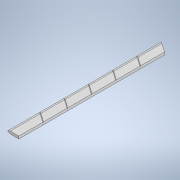
# Autodesk Inventor part: blade a.
Saved by Autodesk Inventor 2021 (Build 250183000, 183)
## iProperties
Created: 2021-03-27
Part Number: blade a.
Material: Generic
Document SubType Name: Modeling
Designer: newic
Density: 1 g/cm^3
Appearance: Default
Author: newic
Autodesk Inventor part; units mm, degrees
ref_plane "YZ Plane" through (0, 0, 0) normal (1, 0, 0) x (0, 1, 0)
ref_plane "XZ Plane" through (0, 0, 0) normal (0, 1, 0) x (-1, 0, 0)
ref_plane "XY Plane" through (0, 0, 0) normal (0, 0, 1) x (1, 0, 0)
sketch "Sketch1" plane through (0, 0, 0) normal (0, 1, 0) x (-1, 0, 0)
  line L0 (0, 0) -> (50.9694, 0)
  line L1 (50.9694, 0) -> (50.9694, -698.5)
  line L2 (0, -662.8108) -> (0, 0)
  line L3 (50.9694, -698.5) -> (133.3543, -698.5) construction
  line L4 (0, -647.5306) -> (0, -662.8108)
  line L5 (0, -662.8108) -> (50.9694, -698.5)
  dimension "d0" = 698.5
  dimension "d10" = 55
  constraints: 12 end point, 2 horizontal, 1 collinear, 1 parallel, 1 perpendicular, 1 point on line
  measures "d0" distance of L0.end L1.end
  measures "d10" angle of L5 L1
extrude "Extrusion1" add sketch "Sketch1" along normal blind 11.43
chamfer "Chamfer1" distance 11.43 angle 22.5 1 edges at (-50.9694, 11.43, -349.25) measured on face at (-33.9796, 11.43, -453.7703)
chamfer "Chamfer2" distance 11.43 angle 22.5 1 edges at (-50.9694, 0, -349.25) measured on face at (-33.9796, 0, -453.7703)
sketch "Sketch2" plane through (0, 11.43, 0) normal (0, 1, 0) x (1, 0, 0)
  line L0 (0, 0) -> (0, 662.8108) projected
  line L1 (0, 662.8108) -> (-39.5394, 690.4966) projected
  line L2 (0, 0) -> (0, 662.8108)
  line L3 (0, 662.8108) -> (0, 552.3208)
  line L4 (0, 552.3208) -> (0, 441.8308)
  line L5 (0, 441.8308) -> (0, 331.3408)
  line L6 (0, 331.3408) -> (0, 220.8508)
  line L7 (0, 220.8508) -> (0, 110.3608)
  line L8 (0, 110.3608) -> (0, -0.1292)
  line L9 (-50.9694, 698.5) -> (-50.9694, 0) projected
  line L10 (0, 552.3208) -> (62.2222, 552.3208) construction
  line L11 (0, 441.8308) -> (75.6755, 441.8308) construction
  line L12 (0, 331.3408) -> (96.3167, 331.3408) construction
  line L13 (0, 220.8508) -> (100.8131, 220.8508) construction
  line L14 (0, 110.3608) -> (129.8585, 110.3608) construction
  line L15 (0.7284, 553.3611) -> (-50.241, 589.0503)
  line L16 (-0.7284, 551.2805) -> (-51.6979, 586.9697)
  line L17 (0.7284, 442.8711) -> (-50.241, 478.5603)
  line L18 (-0.7284, 440.7905) -> (-51.6979, 476.4797)
  line L19 (0.7284, 332.3811) -> (-50.241, 368.0703)
  line L20 (-0.7284, 330.3005) -> (-51.6979, 365.9897)
  line L21 (0.7284, 221.8911) -> (-50.241, 257.5803)
  line L22 (-0.7284, 219.8105) -> (-51.6979, 255.4997)
  line L23 (0.7284, 111.4011) -> (-50.241, 147.0903)
  line L24 (-0.7284, 109.3205) -> (-51.6979, 145.0097)
  line L25 (-55.7095, 150.6945) -> (-51.6979, 145.0097)
  line L26 (6.2736, 109.3205) -> (0.7284, 111.4011)
  line L27 (4.7871, 219.8105) -> (0.7284, 221.8911)
  line L28 (-50.241, 257.5803) -> (-56.0233, 261.6292)
  line L29 (-56.0233, 261.6292) -> (-51.6979, 255.4997)
  line L30 (-0.7284, 109.3205) -> (2.432, 107.1075)
  line L31 (2.432, 107.1075) -> (6.2736, 109.3205)
  line L32 (-50.241, 147.0903) -> (-53.1322, 149.1147)
  line L33 (-53.1322, 149.1147) -> (-55.7095, 150.6945)
  line L34 (-0.7284, 219.8105) -> (1.0647, 218.5549)
  line L35 (1.0647, 218.5549) -> (4.7871, 219.8105)
  line L36 (-0.7284, 330.3005) -> (6.2736, 325.3976)
  line L37 (6.2736, 325.3976) -> (0.7284, 332.3811)
  line L38 (-50.241, 368.0703) -> (-56.0233, 372.1192)
  line L39 (-56.0233, 372.1192) -> (-51.6979, 365.9897)
  line L40 (-0.7284, 440.7905) -> (6.2736, 435.8876)
  line L41 (6.2736, 435.8876) -> (0.7284, 442.8711)
  line L42 (-50.241, 478.5603) -> (-56.4046, 482.8761)
  line L43 (-56.4046, 482.8761) -> (-51.6979, 476.4797)
  line L44 (-0.7284, 551.2805) -> (4.3528, 547.7226)
  line L45 (4.3528, 547.7226) -> (0.7284, 553.3611)
  line L46 (-50.241, 589.0503) -> (-53.8606, 591.5848)
  line L47 (-53.8606, 591.5848) -> (-51.6979, 586.9697)
  dimension "d11" = 110.49
  dimension "d12" = 110.49
  dimension "d13" = 110.49
  dimension "d14" = 110.49
  dimension "d15" = 110.49
  dimension "d16" = 110.49
  constraints: 90 end point, 10 point on line, 8 parallel, 5 horizontal, 1 vertical
  measures "d11" distance of L0.end L3.end
  measures "d12" distance of L3.end L4.end
  measures "d13" distance of L4.end L5.end
  measures "d14" distance of L5.end L6.end
  measures "d15" distance of L6.end L7.end
  measures "d16" distance of L7.end L8.end
sketch "Sketch3" plane through (0, 0, 0) normal (0, -1, 0) x (1, 0, 0)
  line L0 (0, 0) -> (0, 662.8108)
  line L1 (0, 662.8108) -> (-39.5394, 690.4966)
  line L2 (0, 0) -> (0, 662.8108)
  line L3 (0, 662.8108) -> (0, 552.3208)
  line L4 (0, 552.3208) -> (0, 441.8308)
  line L5 (0, 441.8308) -> (0, 331.3408)
  line L6 (0, 331.3408) -> (0, 220.8508)
  line L7 (0, 220.8508) -> (0, 110.3608)
  line L8 (0, 110.3608) -> (0, -0.1292)
  line L9 (-50.9694, 698.5) -> (-50.9694, 0)
  line L10 (0, 552.3208) -> (62.2222, 552.3208) construction
  line L11 (0, 441.8308) -> (75.6755, 441.8308) construction
  line L12 (0, 331.3408) -> (96.3167, 331.3408) construction
  line L13 (0, 220.8508) -> (100.8131, 220.8508) construction
  line L14 (0, 110.3608) -> (129.8585, 110.3608) construction
  line L15 (0.7284, 553.3611) -> (-50.241, 589.0503)
  line L16 (-0.7284, 551.2805) -> (-51.6979, 586.9697)
  line L17 (0.7284, 442.8711) -> (-50.241, 478.5603)
  line L18 (-0.7284, 440.7905) -> (-51.6979, 476.4797)
  line L19 (0.7284, 332.3811) -> (-50.241, 368.0703)
  line L20 (-0.7284, 330.3005) -> (-51.6979, 365.9897)
  line L21 (0.7284, 221.8911) -> (-50.241, 257.5803)
  line L22 (-0.7284, 219.8105) -> (-51.6979, 255.4997)
  line L23 (0.7284, 111.4011) -> (-50.241, 147.0903)
  line L24 (-0.7284, 109.3205) -> (-51.6979, 145.0097)
  line L25 (-55.7095, 150.6945) -> (-51.6979, 145.0097)
  line L26 (6.2736, 109.3205) -> (0.7284, 111.4011)
  line L27 (4.7871, 219.8105) -> (0.7284, 221.8911)
  line L28 (-50.241, 257.5803) -> (-56.0233, 261.6292)
  line L29 (-56.0233, 261.6292) -> (-51.6979, 255.4997)
  line L30 (-0.7284, 109.3205) -> (2.432, 107.1075)
  line L31 (2.432, 107.1075) -> (6.2736, 109.3205)
  line L32 (-50.241, 147.0903) -> (-53.1322, 149.1147)
  line L33 (-53.1322, 149.1147) -> (-55.7095, 150.6945)
  line L34 (-0.7284, 219.8105) -> (1.0647, 218.5549)
  line L35 (1.0647, 218.5549) -> (4.7871, 219.8105)
  line L36 (-0.7284, 330.3005) -> (6.2736, 325.3976)
  line L37 (6.2736, 325.3976) -> (0.7284, 332.3811)
  line L38 (-50.241, 368.0703) -> (-56.0233, 372.1192)
  line L39 (-56.0233, 372.1192) -> (-51.6979, 365.9897)
  line L40 (-0.7284, 440.7905) -> (6.2736, 435.8876)
  line L41 (6.2736, 435.8876) -> (0.7284, 442.8711)
  line L42 (-50.241, 478.5603) -> (-56.4046, 482.8761)
  line L43 (-56.4046, 482.8761) -> (-51.6979, 476.4797)
  line L44 (-0.7284, 551.2805) -> (4.3528, 547.7226)
  line L45 (4.3528, 547.7226) -> (0.7284, 553.3611)
  line L46 (-50.241, 589.0503) -> (-53.8606, 591.5848)
  line L47 (-53.8606, 591.5848) -> (-51.6979, 586.9697)
  line L48 (103.6669, -0.1292) -> (-162.6593, -0.1292)
  line L49 (0, -442.0892) -> (0, -331.5992)
  line L50 (-50.9694, -698.7584) -> (-50.9694, -0.2584)
  line L51 (0, -0.2584) -> (0, -663.0692)
  line L52 (0, -0.2584) -> (0, -663.0692)
  line L53 (0, -331.5992) -> (0, -221.1092)
  line L54 (0, -110.6192) -> (0, -0.1292)
  line L55 (-0.7284, -441.0489) -> (6.2736, -436.146)
  line L56 (6.2736, -436.146) -> (0.7284, -443.1295)
  line L57 (-0.7284, -441.0489) -> (-51.6979, -476.738)
  line L58 (0.7284, -443.1295) -> (-50.241, -478.8187)
  line L59 (-50.241, -478.8187) -> (-56.4046, -483.1345)
  line L60 (-56.4046, -483.1345) -> (-51.6979, -476.738)
  line L61 (0, -552.5792) -> (0, -442.0892)
  line L62 (-0.7284, -551.5389) -> (4.3528, -547.9809)
  line L63 (-0.7284, -551.5389) -> (-51.6979, -587.228)
  line L64 (0.7284, -553.6195) -> (-50.241, -589.3087)
  line L65 (-53.8606, -591.8432) -> (-51.6979, -587.228)
  line L66 (0, -663.0692) -> (-39.5394, -690.755)
  line L67 (4.3528, -547.9809) -> (0.7284, -553.6195)
  line L68 (0, -552.5792) -> (62.2222, -552.5792) construction
  line L69 (0, -663.0692) -> (0, -552.5792)
  line L70 (-50.241, -589.3087) -> (-53.8606, -591.8432)
  line L71 (0, -221.1092) -> (0, -110.6192)
  line L72 (4.7871, -220.0689) -> (0.7284, -222.1495)
  line L73 (-0.7284, -220.0689) -> (1.0647, -218.8133)
  line L74 (1.0647, -218.8133) -> (4.7871, -220.0689)
  line L75 (6.2736, -109.5789) -> (0.7284, -111.6595)
  line L76 (-0.7284, -109.5789) -> (2.432, -107.3659)
  line L77 (2.432, -107.3659) -> (6.2736, -109.5789)
  line L78 (0, -442.0892) -> (75.6755, -442.0892) construction
  line L79 (0, -331.5992) -> (96.3167, -331.5992) construction
  line L80 (-50.241, -368.3287) -> (-56.0233, -372.3775)
  line L81 (0.7284, -332.6395) -> (-50.241, -368.3287)
  line L82 (-0.7284, -330.5589) -> (-51.6979, -366.248)
  line L83 (-0.7284, -330.5589) -> (6.2736, -325.656)
  line L84 (6.2736, -325.656) -> (0.7284, -332.6395)
  line L85 (-56.0233, -372.3775) -> (-51.6979, -366.248)
  line L86 (-0.7284, -109.5789) -> (-51.6979, -145.268)
  line L87 (0.7284, -111.6595) -> (-50.241, -147.3487)
  line L88 (-50.241, -147.3487) -> (-53.1322, -149.3731)
  line L89 (-55.7095, -150.9528) -> (-51.6979, -145.268)
  line L90 (-53.1322, -149.3731) -> (-55.7095, -150.9528)
  line L91 (-0.7284, -220.0689) -> (-51.6979, -255.758)
  line L92 (0.7284, -222.1495) -> (-50.241, -257.8387)
  line L93 (-50.241, -257.8387) -> (-56.0233, -261.8875)
  line L94 (-56.0233, -261.8875) -> (-51.6979, -255.758)
  dimension "d32" = 110.49
  dimension "d33" = 110.49
  dimension "d34" = 110.49
  dimension "d35" = 110.49
  dimension "d36" = 110.49
  dimension "d37" = 110.49
  constraints: 190 end point, 50 symmetric about line, 20 point on line, 8 parallel, 6 horizontal, 1 vertical
  measures "d32" distance of L0.end L4.start
  measures "d33" distance of L4.start L5.start
  measures "d34" distance of L5.start L5.end
  measures "d35" distance of L5.end L6.end
  measures "d36" distance of L6.end L8.start
  measures "d37" distance of L8.start L8.end
extrude "Extrusion2" cut sketch "Sketch2" against normal blind 0.889 contours L30 L24 L9 L32 L23 L0 | L0 L23 L26 L31 L30 | L24 L25 L33 L32 L9 | L34 L22 L9 L28 L21 L0 | L0 L21 L27 L35 L34 | L22 L29 L28 L9 | L36 L20 L9 L38 L19 L0 | L0 L19 L37 L36 | L20 L39 L38 L9 | L18 L43 L42 L9 | L9 L42 L17 L0 L40 L18 | L0 L17 L41 L40 | L16 L47 L46 L9 | L9 L46 L15 L0 L44 L16 | L0 L15 L45 L44
extrude "Extrusion3" cut sketch "Sketch3" against normal blind 0.889 contours L76 L77 L75 L87 L51 | L51 L87 L88 L50 L86 L76 | L50 L88 L90 L89 L86 | L73 L74 L72 L92 L51 | L51 L92 L93 L50 L91 L73 | L50 L93 L94 L91 | L83 L84 L81 L49 L51 | L51 L49 L81 L80 L50 L82 L83 | L50 L80 L85 L82 | L57 L55 L49 L51 L58 L59 L50 | L50 L59 L60 L57 | L55 L56 L58 L51 L49 | L63 L62 L51 L64 L70 L50 | L50 L70 L65 L63 | L62 L67 L64 L51
sketch "Sketch8" plane through (-50.9694, 4.7345, -698.5) normal (-0.3827, -0.9239, 0) x (0.9239, -0.3827, 0)
  line L0 (10.0487, 560.2426) -> (12.3717, 561.7454) projected
  line L1 (12.3717, 561.7454) -> (-8.9548, 547.9491)
  line L2 (12.3717, 558.6446) -> (10.0487, 557.1418) projected
  line L3 (12.3717, 558.6446) -> (-8.9548, 544.8483)
  line L4 (-8.9548, 544.8483) -> (-8.6984, 548.5745)
  line L5 (48.9014, 475.8404) -> (12.3717, 448.1546) projected
  line L6 (12.3717, 448.1546) -> (-8.9548, 434.3583)
  line L7 (12.3717, 448.1546) -> (10.0487, 446.6518) projected
  line L8 (12.3717, 451.2554) -> (12.3717, 558.6446) projected
  line L9 (12.3717, 451.2554) -> (-8.9548, 437.4591)
  line L10 (10.0487, 449.7526) -> (12.3717, 451.2554) projected
  line L11 (12.3717, 340.7654) -> (12.3717, 448.1546) projected
  line L12 (12.3717, 340.7654) -> (-8.9548, 326.9691)
  line L13 (10.0487, 339.2626) -> (12.3717, 340.7654) projected
  line L14 (12.3717, 230.2754) -> (12.3717, 337.6646) projected
  line L15 (12.3717, 337.6646) -> (-8.9548, 323.8683)
  line L16 (12.3717, 230.2754) -> (-8.9548, 216.4791)
  line L17 (10.0487, 228.7726) -> (12.3717, 230.2754) projected
  line L18 (12.3717, 119.7854) -> (12.3717, 227.1746) projected
  line L19 (12.3717, 227.1746) -> (-8.9548, 213.3783)
  line L20 (12.3717, 227.1746) -> (10.0487, 225.6718) projected
  line L21 (12.3717, 119.7854) -> (-8.9548, 105.9891)
  line L22 (12.3717, 8.0034) -> (12.3717, 116.6846) projected
  line L23 (12.3717, 116.6846) -> (-8.9548, 102.8883)
  line L24 (-5.4774, 100.6137) -> (-5.4774, 558.6446)
  line L25 (0, 698.5) -> (0, 0) projected
  line L26 (12.3717, 561.7454) -> (12.3717, 698.5) projected
  line L27 (12.3717, 566.5432) -> (12.3717, 51.1838)
  point P0 (48.9014, 698.5)
  point P1 (12.3717, 561.7454)
  point P2 (-5.4774, 550.1987)
  point P3 (-5.4774, 547.0979)
  point P4 (12.3717, 448.1546)
  point P5 (-5.4774, 439.7087)
  point P6 (-5.4774, 436.6079)
  point P7 (-5.4774, 218.7287)
  point P8 (-5.4774, 215.6279)
  point P9 (-5.4774, 108.2387)
  point P10 (-5.4774, 105.1379)
  point P11 (-5.4774, 329.2187)
  point P12 (-5.4774, 326.1179)
  dimension "d42" = 25.4
  dimension "d43" = 25.4
  dimension "d44" = 25.4
  dimension "d45" = 25.4
  dimension "d46" = 25.4
  dimension "d47" = 25.4
  dimension "d48" = 25.4
  dimension "d49" = 25.4
  dimension "d50" = 25.4
  dimension "d51" = 25.4
  constraints: 26 end point, 6 collinear, 2 point on line, 1 parallel
  measures "d42" distance of L0.end L1.end
  measures "d43" distance of L2.start L3.end
  measures "d44" distance of L5.end L6.end
  measures "d45" distance of L8.start L9.end
  measures "d46" distance of L11.start L12.end
  measures "d47" distance of L14.end L15.end
  measures "d48" distance of L14.start L16.end
  measures "d49" distance of L18.end L19.end
  measures "d50" distance of L18.start L21.end
  measures "d51" distance of L22.end L23.end
extrude "Extrusion4" cut sketch "Sketch8" against normal blind 0.889 contours L0 L27 L2 L3 L25 L1 | L25 L3 L24 L1 | L27 L6 L25 L9 | L25 L6 L24 L9 | L27 L15 L25 L12 | L25 L15 L24 L12 | L27 L19 L25 L16 | L25 L19 L24 L16 | L27 L23 L25 L21 | L25 L23 L24 L21
sketch "Sketch9" plane through (-50.9694, 6.6955, 0) normal (-0.3827, 0.9239, 0) x (0.9239, 0.3827, 0)
  line L0 (12.3717, 0) -> (12.3717, 136.4962) projected
  line L1 (12.3717, 136.4962) -> (-8.9576, 150.2883)
  line L2 (12.3717, 139.597) -> (12.3717, 246.9862) projected
  line L3 (12.3717, 139.597) -> (-8.9548, 153.3933)
  line L4 (10.0487, 141.0998) -> (12.3717, 139.597) projected
  line L5 (12.3717, 246.9862) -> (10.0487, 248.4891) projected
  line L6 (12.3717, 246.9862) -> (-8.9548, 260.7826)
  line L7 (12.3717, 250.087) -> (12.3717, 357.4762) projected
  line L8 (12.3717, 250.087) -> (-8.9548, 263.8833)
  line L9 (10.0487, 251.5898) -> (12.3717, 250.087) projected
  line L10 (12.3717, 357.4762) -> (10.0487, 358.9791) projected
  line L11 (12.3717, 357.4762) -> (-8.9548, 371.2726)
  line L12 (10.0487, 362.0798) -> (12.3717, 360.577) projected
  line L13 (12.3717, 360.577) -> (-8.9548, 374.3733)
  line L14 (12.3717, 467.9662) -> (10.0487, 469.4691) projected
  line L15 (12.3717, 467.9662) -> (-8.9548, 481.7626)
  line L16 (12.3717, 471.067) -> (-8.9548, 484.8633)
  line L17 (10.0487, 472.5698) -> (12.3717, 471.067) projected
  line L18 (12.3717, 578.4562) -> (10.0487, 579.9591) projected
  line L19 (12.3717, 578.4562) -> (-8.9548, 592.2526)
  line L20 (10.0487, 583.0598) -> (12.3717, 581.557) projected
  line L21 (12.3717, 581.557) -> (-8.9548, 595.3533)
  line L22 (12.3717, 581.557) -> (12.3717, 690.4966) projected
  line L23 (12.3717, 590.3666) -> (12.3717, 104.1436)
  line L24 (-2.7877, 113.0522) -> (-2.7877, 598.5214)
  point P0 (44.5273, 0)
  point P1 (-2.7877, 591.3638)
  point P2 (-2.7877, 588.263)
  point P3 (12.3717, 578.4562)
  point P4 (12.3717, 581.557)
  point P5 (-2.7877, 480.8738)
  point P6 (-2.7877, 477.773)
  point P7 (12.3717, 471.067)
  point P8 (-2.7877, 370.3838)
  point P9 (-2.7877, 367.283)
  point P10 (12.3717, 357.4762)
  point P11 (-2.7877, 259.8938)
  point P12 (-2.7877, 256.793)
  point P13 (-2.7877, 149.4038)
  point P14 (-2.7877, 146.2987)
  dimension "d54" = 25.4
  dimension "d55" = 25.4
  dimension "d56" = 25.4
  dimension "d57" = 25.4
  dimension "d58" = 25.4
  dimension "d59" = 25.4
  dimension "d60" = 25.4
  dimension "d61" = 25.4
  dimension "d62" = 25.4
  dimension "d63" = 25.4
  constraints: 24 end point, 7 collinear, 2 point on line, 1 vertical
  measures "d54" distance of L0.end L1.end
  measures "d55" distance of L2.start L3.end
  measures "d56" distance of L2.end L6.end
  measures "d57" distance of L7.start L8.end
  measures "d58" distance of L7.end L11.end
  measures "d59" distance of L12.end L13.end
  measures "d60" distance of L14.start L15.end
  measures "d61" distance of L16.start L16.end
  measures "d62" distance of L18.start L19.end
  measures "d63" distance of L20.end L21.end
extrude "Extrusion5" cut sketch "Sketch9" against normal blind 0.889 contours L1 L24 L3 L23 | L5 L6 L24 L8 L23 | L10 L11 L24 L13 L12 L23 | L14 L15 L24 L16 L23 | L18 L19 L24 L21 L20 L23
body "Solid1"
